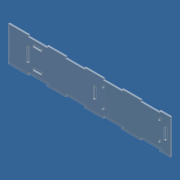
# Autodesk Inventor part: Bottom
Saved by Autodesk Inventor 2016 (Build 200138000, 138)
## iProperties
Created: 2016-04-03
Part Number: Bottom
Material: Polycarbonate, Clear
Document SubType Name: Modeling
Designer: admin
Density: 1.2 g/cm^3
Appearance: Polycarbonate - Clear
Author: admin
Autodesk Inventor part; units mm, degrees
ref_plane "YZ Plane" through (0, 0, 0) normal (1, 0, 0) x (0, 1, 0)
ref_plane "XZ Plane" through (0, 0, 0) normal (0, 1, 0) x (-1, 0, 0)
ref_plane "XY Plane" through (0, 0, 0) normal (0, 0, 1) x (1, 0, 0)
derived "Wall.ipt"
sketch "Sketch1" plane through (0, 0, 0) normal (0, 0, 1) x (1, 0, 0)
  line L0 (142.5, -22.5) -> (142.5, 22.5)
  arc A0 (-169.3198, -9.3198) -> (-157.5, -22.5) centre (-130.5627, 13.547) ccw
  line L1 (-154.4706, 5.5294) -> (-150.935, 1.9939)
  line L2 (-150.935, 1.9939) -> (-152.2157, 0.7132)
  line L3 (-152.2157, 0.7132) -> (-150.8015, -0.701)
  line L4 (-150.8015, -0.701) -> (-149.5208, 0.5797)
  line L5 (-149.5208, 0.5797) -> (-147.3995, -1.5416)
  line L6 (-147.3995, -1.5416) -> (-145.2782, 0.5797)
  line L7 (-145.2782, 0.5797) -> (-147.3995, 2.701)
  line L8 (-147.3995, 2.701) -> (-146.1188, 3.9817)
  line L9 (-146.1188, 3.9817) -> (-147.533, 5.3959)
  line L10 (-147.533, 5.3959) -> (-148.8137, 4.1152)
  line L11 (-148.8137, 4.1152) -> (-152.3492, 7.6508)
  line L12 (-154.542, 7.7222) -> (-156.666, 9.8462) construction
  line L13 (-122.5, 22.5) -> (-122.5, 25.5)
  line L14 (-122.5, 25.5) -> (-87.5, 25.5)
  line L15 (-87.5, 25.5) -> (-87.5, 22.5)
  line L16 (-52.5, 22.5) -> (-52.5, 25.5)
  line L17 (-52.5, 25.5) -> (-17.5, 25.5)
  line L18 (-17.5, 25.5) -> (-17.5, 22.5)
  line L19 (17.5, 22.5) -> (17.5, 25.5)
  line L20 (17.5, 25.5) -> (52.5, 25.5)
  line L21 (52.5, 25.5) -> (52.5, 22.5)
  line L22 (87.5, 22.5) -> (87.5, 25.5)
  line L23 (87.5, 25.5) -> (122.5, 25.5)
  line L24 (122.5, 25.5) -> (122.5, 22.5)
  line L25 (87.5, 22.5) -> (52.5, 22.5)
  line L26 (-52.5, 22.5) -> (-87.5, 22.5)
  line L27 (-122.5, 22.5) -> (-137.5, 22.5)
  line L28 (-122.5, -22.5) -> (-122.5, -25.5)
  line L29 (-122.5, -25.5) -> (-87.5, -25.5)
  line L30 (-87.5, -25.5) -> (-87.5, -22.5)
  line L31 (-52.5, -22.5) -> (-52.5, -25.5)
  line L32 (-52.5, -25.5) -> (-17.5, -25.5)
  line L33 (-17.5, -25.5) -> (-17.5, -22.5)
  line L34 (17.5, -22.5) -> (17.5, -25.5)
  line L35 (17.5, -25.5) -> (52.5, -25.5)
  line L36 (52.5, -25.5) -> (52.5, -22.5)
  line L37 (87.5, -22.5) -> (87.5, -25.5)
  line L38 (87.5, -25.5) -> (122.5, -25.5)
  line L39 (122.5, -25.5) -> (122.5, -22.5)
  line L40 (-157.5, -22.5) -> (-122.5, -22.5)
  line L41 (-87.5, -22.5) -> (-52.5, -22.5)
  line L42 (-17.5, -22.5) -> (17.5, -22.5)
  line L43 (52.5, -22.5) -> (87.5, -22.5)
  line L44 (122.5, -22.5) -> (142.5, -22.5)
  line L45 (-1.5, 12.5) -> (-1.5, 22.5)
  line L46 (1.5, 22.5) -> (1.5, 12.5)
  line L47 (1.5, 12.5) -> (-1.5, 12.5)
  line L48 (-37.337, 0) -> (-30.889, 0) construction
  line L49 (-164.0165, -4.0165) -> (-166.1378, -1.8952)
  line L50 (-166.1378, -1.8952) -> (-161.8952, 2.3475)
  line L51 (-161.8952, 2.3475) -> (-159.7739, 0.2261)
  line L52 (-147.0459, 12.9541) -> (-149.1673, 15.0754)
  line L53 (-149.1673, 15.0754) -> (-144.9246, 19.318)
  line L54 (-144.9246, 19.318) -> (-142.8033, 17.1967)
  line L55 (-154.4706, 5.5294) -> (-159.7739, 0.2261)
  line L56 (-164.0165, -4.0165) -> (-169.3198, -9.3198)
  line L57 (-137.5, 22.5) -> (-142.8033, 17.1967)
  line L58 (-147.0459, 12.9541) -> (-152.3492, 7.6508)
  line L59 (17.5, 22.5) -> (1.5, 22.5)
  line L60 (-1.5, 22.5) -> (-17.5, 22.5)
  line L61 (131, 22.5) -> (131, 12.5)
  line L62 (131, 12.5) -> (134, 12.5)
  line L63 (134, 12.5) -> (134, 22.5)
  line L64 (122.5, 22.5) -> (131, 22.5)
  line L65 (134, 22.5) -> (142.5, 22.5)
  point P0 (0, 0)
  point P1 (142.5, 0)
  point P2 (-159.77, -22.5)
  point P3 (-146.3388, -0.481)
  point P4 (2.493, 0)
  point P5 (0, -22.5)
  point P6 (1.5, -22.5)
sketch "Sketch2" plane through (0, 0, 0) normal (0, 1, 0) x (-1, 0, 0)
  line L0 (-142.5, 0) -> (-142.5, -65)
  line L1 (-142.5, 0) -> (-122.5, 0)
  line L2 (-122.5, 0) -> (-122.5, -3)
  line L3 (-122.5, -3) -> (-87.5, -3)
  line L4 (-87.5, -3) -> (-87.5, 0)
  line L5 (-87.5, 0) -> (-52.5, 0)
  line L6 (-52.5, 0) -> (-52.5, -3)
  line L7 (-52.5, -3) -> (-17.5, -3)
  line L8 (-17.5, -3) -> (-17.5, 0)
  line L9 (-17.5, 0) -> (17.5, 0)
  line L10 (17.5, 0) -> (17.5, -3)
  line L11 (17.5, -3) -> (52.5, -3)
  line L12 (52.5, -3) -> (52.5, 0)
  line L13 (52.5, 0) -> (87.5, 0)
  line L14 (87.5, 0) -> (87.5, -3)
  line L15 (87.5, -3) -> (122.5, -3)
  line L16 (122.5, -3) -> (122.5, 0)
  line L17 (122.5, 0) -> (159.77, 0)
  line L18 (159.77, 0) -> (159.77, -65)
  line L19 (159.77, -65) -> (122.5, -65)
  line L20 (122.5, -65) -> (122.5, -62)
  line L21 (122.5, -62) -> (87.5, -62)
  line L22 (87.5, -62) -> (87.5, -65)
  line L23 (87.5, -65) -> (52.5, -65)
  line L24 (52.5, -65) -> (52.5, -62)
  line L25 (17.5, -62) -> (17.5, -65)
  line L26 (17.5, -62) -> (52.5, -62)
  line L27 (17.5, -65) -> (-17.5, -65)
  line L28 (-17.5, -65) -> (-17.5, -62)
  line L29 (-17.5, -62) -> (-52.5, -62)
  line L30 (-52.5, -62) -> (-52.5, -65)
  line L31 (-52.5, -65) -> (-87.5, -65)
  line L32 (-87.5, -65) -> (-87.5, -62)
  line L33 (-87.5, -62) -> (-122.5, -62)
  line L34 (-122.5, -62) -> (-122.5, -65)
  line L35 (-122.5, -65) -> (-142.5, -65)
  point P0 (0, 0)
  point P1 (0, 0)
  point P2 (159.77, -32.5)
  dimension "d1" = 65
  dimension "d2" = 3
  constraints: 72 end point, 36 point on line, 16 perpendicular, 2 horizontal, 2 midpoint, 1 collinear, 1 vertical
  measures "d1" distance of L0.start L0.end
  measures "d2" distance of L33.end L34.end
extrude "Extrusion1" add sketch "Sketch2" along normal blind 3
sketch "Sketch3" plane through (0, 3, 0) normal (0, 1, 0) x (1, 0, 0)
  line L0 (-125.5, 45) -> (-122.5, 45)
  line L1 (-122.5, 45) -> (-122.5, 20)
  line L2 (-122.5, 20) -> (-125.5, 20)
  line L3 (-125.5, 20) -> (-125.5, 45)
  line L4 (-159.77, 0) -> (-122.5, 0) projected
  line L5 (-122.5, 0) -> (-122.5, 3) projected
  line L6 (-122.5, 3) -> (-87.5, 3) projected
  line L7 (-87.5, 3) -> (-87.5, 0) projected
  line L8 (-87.5, 0) -> (-52.5, 0) projected
  line L9 (-52.5, 0) -> (-52.5, 3) projected
  line L10 (-52.5, 3) -> (-17.5, 3) projected
  line L11 (-17.5, 3) -> (-17.5, 0) projected
  line L12 (-17.5, 0) -> (17.5, 0) projected
  line L13 (17.5, 0) -> (17.5, 3) projected
  line L14 (17.5, 3) -> (52.5, 3) projected
  line L15 (52.5, 3) -> (52.5, 0) projected
  line L16 (52.5, 0) -> (87.5, 0) projected
  line L17 (87.5, 0) -> (87.5, 3) projected
  line L18 (87.5, 3) -> (122.5, 3) projected
  line L19 (122.5, 3) -> (122.5, 0) projected
  line L20 (122.5, 0) -> (142.5, 0) projected
  line L21 (142.5, 0) -> (142.5, 65) projected
  line L22 (142.5, 65) -> (122.5, 65) projected
  line L23 (122.5, 65) -> (122.5, 62) projected
  line L24 (122.5, 62) -> (87.5, 62) projected
  line L25 (87.5, 62) -> (87.5, 65) projected
  line L26 (87.5, 65) -> (52.5, 65) projected
  line L27 (52.5, 65) -> (52.5, 62) projected
  line L28 (52.5, 62) -> (17.5, 62) projected
  line L29 (17.5, 62) -> (17.5, 65) projected
  line L30 (17.5, 65) -> (-17.5, 65) projected
  line L31 (-17.5, 65) -> (-17.5, 62) projected
  line L32 (-17.5, 62) -> (-52.5, 62) projected
  line L33 (-52.5, 62) -> (-52.5, 65) projected
  line L34 (-52.5, 65) -> (-87.5, 65) projected
  line L35 (-87.5, 65) -> (-87.5, 62) projected
  line L36 (-87.5, 62) -> (-122.5, 62) projected
  line L37 (-122.5, 62) -> (-122.5, 65) projected
  line L38 (-122.5, 65) -> (-159.77, 65) projected
  line L39 (-159.77, 65) -> (-159.77, 0) projected
  line L40 (-122.5, 0) -> (-122.5, 3) projected
  line L41 (-114, 53) -> (-99, 53)
  line L42 (-99, 53) -> (-99, 50)
  line L43 (-99, 50) -> (-114, 50)
  line L44 (-114, 50) -> (-114, 53)
  line L45 (-114, 15) -> (-99, 15)
  line L46 (-99, 15) -> (-99, 12)
  line L47 (-99, 12) -> (-114, 12)
  line L48 (-114, 12) -> (-114, 15)
  line L49 (-101.3344, 32.5) -> (-72.214, 32.5) construction
  line L50 (-159.77, 65) -> (-159.77, 0) construction
  line L51 (131, 42.5) -> (134, 42.5)
  line L52 (134, 42.5) -> (134, 22.5)
  line L53 (134, 22.5) -> (131, 22.5)
  line L54 (131, 22.5) -> (131, 42.5)
  line L55 (-1.5, 42.5) -> (1.5, 42.5)
  line L56 (1.5, 42.5) -> (1.5, 22.5)
  line L57 (1.5, 22.5) -> (-1.5, 22.5)
  line L58 (-1.5, 22.5) -> (-1.5, 42.5)
  line L59 (17.5, 62) -> (17.5, 65) projected
  point P0 (0, 0)
  point P1 (-122.5, 32.5)
  point P2 (-159.77, 32.5)
  point P3 (-159.77, 32.5)
  point P4 (1.5, 0)
  point P5 (1.5, 32.5)
  dimension "d5" = 25
  dimension "d6" = 265
  dimension "d9" = 15
  dimension "d10" = 35
  dimension "d11" = 8.5
  dimension "d12" = 8.5
  dimension "d14" = 20
  constraints: 42 end point, 10 parallel, 6 equal length, 6 horizontal, 5 perpendicular, 4 midpoint, 3 point on line, 2 collinear, 1 horizontal alignment, 2 other
  measures "d5" distance of L2.end L0.start
  measures "d6" distance between parallel lines of L21 L1
  measures "d9" distance of L41.start L41.end
  measures "d10" distance between parallel lines of L45 L43
  measures "d11" distance between parallel lines of L44 L1
  measures "d12" distance between parallel lines of L21 L52
  measures "d14" distance between parallel lines of L57 L55
extrude "Extrusion2" cut sketch "Sketch3" against normal blind 3 contours L0 L1 L2 L3 | L41 L42 L43 L44 | L45 L46 L47 L48 | L51 L52 L53 L54 | L55 L56 L57 L58
sketch "Sketch4" plane through (0, 3, 0) normal (0, 1, 0) x (1, 0, 0)
  line L0 (1.5, 42.5) -> (1.5, 22.5) projected
  line L1 (8.604, 32.5) -> (22.5323, 32.5) construction
  point P0 (0, 0)
  point P1 (16.5, 50)
  point P2 (16.5, 15)
  point P3 (121.5, 50)
  point P4 (121.5, 15)
  point P5 (1.5, 32.5)
  dimension "d15" = 35
  dimension "d16" = 15
  dimension "d17" = 105
  constraints: 2 end point, 2 horizontal alignment, 2 vertical alignment, 1 horizontal, 1 midpoint, 1 point on line, 1 symmetric about line
  measures "d15" distance of point (16.5, 15) point (16.5, 50)
  measures "d16" distance from line of point (16.5, 50) L0
  measures "d17" distance of point (121.5, 50) point (16.5, 50)
hole "Hole1" at (16.5, 3, -50) at (16.5, 3, -15) at (121.5, 3, -50) at (121.5, 3, -15) direction (0, -1, 0) diameter 3 end through all countersink diameter 5 countersink angle 90
body "Solid1"
